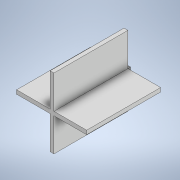
# Autodesk Inventor part: Gitter
Saved by Autodesk Inventor 2020 (Build 240168000, 168)
## iProperties
Created: 2021-05-12
Part Number: Gitter
Material: Generisch
Document SubType Name: Modeling
Designer: Julian Uhl
Density: 1 g/cm^3
Appearance: Vorgabe
Author: Julian Uhl
Autodesk Inventor part; units mm, degrees
ref_plane "YZ Plane" through (0, 0, 0) normal (1, 0, 0) x (0, 1, 0)
ref_plane "XZ Plane" through (0, 0, 0) normal (0, 1, 0) x (-1, 0, 0)
ref_plane "XY Plane" through (0, 0, 0) normal (0, 0, 1) x (1, 0, 0)
sketch "Skizze1" plane through (0, 0, 0) normal (0, 0, 1) x (1, 0, 0)
  line L0 (-126, 0) -> (126, 0) projected
  line L1 (0, -126) -> (0, 126) projected
  line L2 (-90, 4.7809) -> (90, 4.7809)
  line L3 (90, 4.7809) -> (90, -5.2191)
  line L4 (90, -5.2191) -> (-90, -5.2191)
  line L5 (-90, -5.2191) -> (-90, 4.7809)
  line L6 (-4.0898, 90) -> (5.9102, 90)
  line L7 (5.9102, 90) -> (5.9102, -90)
  line L8 (5.9102, -90) -> (-4.0898, -90)
  line L9 (-4.0898, -90) -> (-4.0898, 90)
  point P0 (0, 0)
  point P1 (-4.0898, 4.7809)
  point P2 (-4.0898, -5.2191)
  point P3 (5.9102, -5.2191)
  point P4 (5.9102, 4.7809)
  dimension "d0" = 10
  dimension "d1" = 180
  dimension "d2" = 90
  dimension "d3" = 10
  dimension "d4" = 180
  dimension "d5" = 90
  constraints: 16 end point, 4 parallel, 2 horizontal, 2 perpendicular
  measures "d0" distance between parallel lines of L4 L2
  measures "d1" distance between parallel lines of L3 L5
  measures "d2" distance between parallel lines of L1 L5
  measures "d3" distance between parallel lines of L7 L9
  measures "d4" distance between parallel lines of L8 L6
  measures "d5" distance between parallel lines of L0 L8
extrude "Extrusion1" add sketch "Skizze1" along normal blind 190
sketch "Skizze2" plane through (0, 0, 0) normal (0, 0, -1) x (-1, 0, 0)
  line L0 (-90, 4.7809) -> (-5.9102, 4.7809) projected
  line L1 (90, -5.2191) -> (4.0898, -5.2191) projected
  line L2 (-5.9102, 4.7809) -> (4.0898, 4.7809)
  line L3 (4.0898, 4.7809) -> (4.0898, -5.2191)
  line L4 (4.0898, -5.2191) -> (-5.9102, -5.2191)
  line L5 (-5.9102, -5.2191) -> (-5.9102, 4.7809)
  point P0 (0, 0)
  constraints: 8 end point, 2 parallel, 1 horizontal, 1 perpendicular
extrude "Extrusion2" add sketch "Skizze2" along normal blind 7
